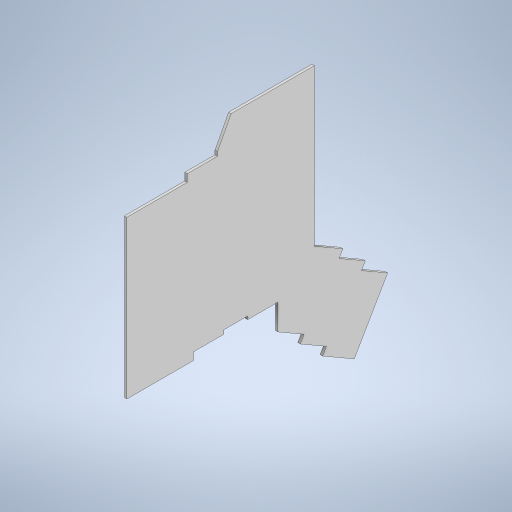
# Autodesk Inventor part: board-profile
Saved by Autodesk Inventor 2024.1 (Build 281209000, 209)
## iProperties
Created: 2023-11-07
Part Number: board-profile
Material: Générique
Document SubType Name: Modeling
Designer: Thibault
Density: 1 g/cm^3
Appearance: Par défaut
Author: Thibault
Autodesk Inventor part; units mm, degrees
ref_plane "YZ Plane" through (0, 0, 0) normal (1, 0, 0) x (0, 1, 0)
ref_plane "XZ Plane" through (0, 0, 0) normal (0, 1, 0) x (-1, 0, 0)
ref_plane "XY Plane" through (0, 0, 0) normal (0, 0, 1) x (1, 0, 0)
sketch "Key" plane through (0, 0, 0) normal (0, 0, 1) x (1, 0, 0)
  line L0 (-9.525, 9.525) -> (9.525, 9.525) construction
  line L1 (9.525, 9.525) -> (9.525, -9.525) construction
  line L2 (9.525, -9.525) -> (-9.525, -9.525) construction
  line L3 (-9.525, -9.525) -> (-9.525, 9.525) construction
  line L4 (-9.525, 9.525) -> (9.525, -9.525) construction
  line L5 (9.525, 9.525) -> (-9.525, -9.525) construction
  point P0 (0, 0)
  point P1 (0, 0)
  dimension "d6" = 19.05
  dimension "d7" = 19.05
  measures "d6" distance of L1.end L2.end
  measures "d7" distance of L0.end L1.end
sketch "Col5" plane through (0, 0, 0) normal (0, 0, 1) x (1, 0, 0)
  line L0 (8.1849, 9.525) -> (27.2349, 9.525) construction
  line L1 (27.2349, 9.525) -> (27.2349, -9.525) construction
  line L2 (27.2349, -9.525) -> (8.1849, -9.525) construction
  line L3 (8.1849, -9.525) -> (8.1849, 9.525) construction
  line L4 (8.1849, 9.525) -> (27.2349, -9.525) construction
  line L5 (27.2349, 9.525) -> (8.1849, -9.525) construction
  line L6 (-10.8651, 9.525) -> (8.1849, 9.525) construction
  line L7 (8.1849, 9.525) -> (8.1849, -9.525) construction
  line L8 (8.1849, -9.525) -> (-10.8651, -9.525) construction
  line L9 (-10.8651, -9.525) -> (-10.8651, 9.525) construction
  line L10 (-10.8651, 9.525) -> (8.1849, -9.525) construction
  line L11 (8.1849, 9.525) -> (-10.8651, -9.525) construction
  line L12 (-29.9151, 9.525) -> (-10.8651, 9.525) construction
  line L13 (-10.8651, 9.525) -> (-10.8651, -9.525) construction
  line L14 (-10.8651, -9.525) -> (-29.9151, -9.525) construction
  line L15 (-29.9151, -9.525) -> (-29.9151, 9.525) construction
  line L16 (-29.9151, 9.525) -> (-10.8651, -9.525) construction
  line L17 (-10.8651, 9.525) -> (-29.9151, -9.525) construction
  line L18 (-48.9651, 9.525) -> (-29.9151, 9.525) construction
  line L19 (-29.9151, 9.525) -> (-29.9151, -9.525) construction
  line L20 (-29.9151, -9.525) -> (-48.9651, -9.525) construction
  line L21 (-48.9651, -9.525) -> (-48.9651, 9.525) construction
  line L22 (-48.9651, 9.525) -> (-29.9151, -9.525) construction
  line L23 (-29.9151, 9.525) -> (-48.9651, -9.525) construction
  line L24 (27.2349, 9.525) -> (46.2849, 9.525) construction
  line L25 (46.2849, 9.525) -> (46.2849, -9.525) construction
  line L26 (46.2849, -9.525) -> (27.2349, -9.525) construction
  line L27 (27.2349, -9.525) -> (27.2349, 9.525) construction
  line L28 (27.2349, 9.525) -> (46.2849, -9.525) construction
  line L29 (46.2849, 9.525) -> (27.2349, -9.525) construction
  point P0 (-10.8651, 0)
sketch "Col4" plane through (0, 0, 0) normal (0, 0, 1) x (1, 0, 0)
  line L0 (8.1849, 9.525) -> (27.2349, 9.525) construction
  line L1 (27.2349, 9.525) -> (27.2349, -9.525) construction
  line L2 (27.2349, -9.525) -> (8.1849, -9.525) construction
  line L3 (8.1849, -9.525) -> (8.1849, 9.525) construction
  line L4 (8.1849, 9.525) -> (27.2349, -9.525) construction
  line L5 (27.2349, 9.525) -> (8.1849, -9.525) construction
  line L6 (-10.8651, 9.525) -> (8.1849, 9.525) construction
  line L7 (8.1849, 9.525) -> (8.1849, -9.525) construction
  line L8 (8.1849, -9.525) -> (-10.8651, -9.525) construction
  line L9 (-10.8651, -9.525) -> (-10.8651, 9.525) construction
  line L10 (-10.8651, 9.525) -> (8.1849, -9.525) construction
  line L11 (8.1849, 9.525) -> (-10.8651, -9.525) construction
  line L12 (-29.9151, 9.525) -> (-10.8651, 9.525) construction
  line L13 (-10.8651, 9.525) -> (-10.8651, -9.525) construction
  line L14 (-10.8651, -9.525) -> (-29.9151, -9.525) construction
  line L15 (-29.9151, -9.525) -> (-29.9151, 9.525) construction
  line L16 (-29.9151, 9.525) -> (-10.8651, -9.525) construction
  line L17 (-10.8651, 9.525) -> (-29.9151, -9.525) construction
  line L18 (-48.9651, 9.525) -> (-29.9151, 9.525) construction
  line L19 (-29.9151, 9.525) -> (-29.9151, -9.525) construction
  line L20 (-29.9151, -9.525) -> (-48.9651, -9.525) construction
  line L21 (-48.9651, -9.525) -> (-48.9651, 9.525) construction
  line L22 (-48.9651, 9.525) -> (-29.9151, -9.525) construction
  line L23 (-29.9151, 9.525) -> (-48.9651, -9.525) construction
  point P0 (-10.8651, 0)
sketch "TC" plane through (0, 0, 0) normal (0, 0, 1) x (1, 0, 0)
  line L0 (-14.8187, 190.1917) -> (1.679, 180.6667) construction
  line L1 (1.679, 180.6667) -> (-7.846, 164.1689) construction
  line L2 (-7.846, 164.1689) -> (-24.3437, 173.6939) construction
  line L3 (-24.3437, 173.6939) -> (-14.8187, 190.1917) construction
  line L4 (-14.8187, 190.1917) -> (-7.846, 164.1689) construction
  line L5 (1.679, 180.6667) -> (-24.3437, 173.6939) construction
  line L6 (-31.3165, 199.7167) -> (-14.8187, 190.1917) construction
  line L7 (-14.8187, 190.1917) -> (-24.3437, 173.6939) construction
  line L8 (-24.3437, 173.6939) -> (-40.8415, 183.2189) construction
  line L9 (-40.8415, 183.2189) -> (-31.3165, 199.7167) construction
  line L10 (-31.3165, 199.7167) -> (-24.3437, 173.6939) construction
  line L11 (-14.8187, 190.1917) -> (-40.8415, 183.2189) construction
  line L12 (-28.4682, 176.0751) -> (-11.9704, 166.5501) construction
  line L13 (-11.9704, 166.5501) -> (-21.4954, 150.0524) construction
  line L14 (-21.4954, 150.0524) -> (-37.9932, 159.5774) construction
  line L15 (-37.9932, 159.5774) -> (-28.4682, 176.0751) construction
  line L16 (-28.4682, 176.0751) -> (-21.4954, 150.0524) construction
  line L17 (-11.9704, 166.5501) -> (-37.9932, 159.5774) construction
  line L18 (-44.966, 185.6001) -> (-28.4682, 176.0751) construction
  line L19 (-28.4682, 176.0751) -> (-37.9932, 159.5774) construction
  line L20 (-37.9932, 159.5774) -> (-54.491, 169.1024) construction
  line L21 (-54.491, 169.1024) -> (-44.966, 185.6001) construction
  line L22 (-44.966, 185.6001) -> (-37.9932, 159.5774) construction
  line L23 (-28.4682, 176.0751) -> (-54.491, 169.1024) construction
  line L24 (-42.1176, 161.9586) -> (-25.6199, 152.4336) construction
  line L25 (-25.6199, 152.4336) -> (-35.1449, 135.9358) construction
  line L26 (-35.1449, 135.9358) -> (-51.6426, 145.4608) construction
  line L27 (-51.6426, 145.4608) -> (-42.1176, 161.9586) construction
  line L28 (-42.1176, 161.9586) -> (-35.1449, 135.9358) construction
  line L29 (-25.6199, 152.4336) -> (-51.6426, 145.4608) construction
  line L30 (-58.6154, 171.4836) -> (-42.1176, 161.9586) construction
  line L31 (-42.1176, 161.9586) -> (-51.6426, 145.4608) construction
  line L32 (-51.6426, 145.4608) -> (-68.1404, 154.9858) construction
  line L33 (-68.1404, 154.9858) -> (-58.6154, 171.4836) construction
  line L34 (-58.6154, 171.4836) -> (-51.6426, 145.4608) construction
  line L35 (-42.1176, 161.9586) -> (-68.1404, 154.9858) construction
  point P0 (-22.1335, 152.0917)
  dimension "d12" = 4.7625
  dimension "d13" = 4.7625
  dimension "d14" = 19.6363
sketch "Esquisse1" plane through (0, 0, 0) normal (1, 0, 0) x (0, 1, 0)
  line L0 (28.177, -71.755) -> (10.397, -71.755) construction
  line L1 (10.397, -71.755) -> (10.397, -102.235) construction
  line L2 (10.397, -102.235) -> (28.177, -102.235)
  line L3 (28.177, -102.235) -> (28.177, -71.755) construction
  line L4 (28.177, -71.755) -> (10.397, -102.235) construction
  line L5 (10.397, -71.755) -> (28.177, -102.235) construction
  line L6 (6.445, 14.065) -> (-92.805, 14.065)
  line L7 (6.445, 14.065) -> (6.445, -24.035)
  line L8 (-68.4861, -104.235) -> (30.177, -104.235)
  line L9 (30.177, -51.755) -> (30.177, -104.235)
  line L10 (-106.1694, -150.4545) -> (-142.6291, -129.4045)
  line L11 (-103.8052, -81.2096) -> (-113.3302, -97.7073)
  line L12 (-113.3302, -97.7073) -> (-117.4547, -95.3261)
  line L13 (-117.4547, -95.3261) -> (-126.9797, -111.8239)
  line L14 (-126.9797, -111.8239) -> (-131.1041, -109.4426)
  line L15 (-131.1041, -109.4426) -> (-142.6291, -129.4045)
  line L16 (-68.4861, -104.235) -> (-78.8706, -122.2214)
  line L17 (-78.8706, -122.2214) -> (-82.995, -119.8402)
  line L18 (-82.995, -119.8402) -> (-92.52, -136.338)
  line L19 (-92.52, -136.338) -> (-96.6444, -133.9567)
  line L20 (-96.6444, -133.9567) -> (-106.1694, -150.4545)
  line L21 (-92.805, 14.065) -> (-92.805, -28.035)
  line L22 (-92.805, -28.035) -> (-88.042, -28.035)
  line L23 (-88.042, -28.035) -> (-88.042, -47.085)
  line L24 (-88.042, -47.085) -> (-85.565, -47.085)
  line L25 (-85.565, -47.085) -> (-85.565, -62.135)
  line L26 (-85.565, -62.135) -> (-87.565, -62.135)
  line L27 (-89.5164, -89.4592) -> (-103.8052, -81.2096) construction
  line L28 (6.445, -24.035) -> (11.208, -24.035)
  line L29 (11.208, -24.035) -> (11.208, -43.085)
  line L30 (11.208, -43.085) -> (13.685, -43.085)
  line L31 (30.177, -51.755) -> (13.685, -43.085)
  line L32 (-78.8706, -122.2214) -> (-92.52, -136.338) construction
  line L33 (-92.52, -136.338) -> (-106.1694, -150.4545) construction
  line L34 (-103.8052, -81.2096) -> (-117.4547, -95.3261) construction
  line L35 (-131.1041, -109.4426) -> (-117.4547, -95.3261) construction
  line L36 (-103.8052, -81.2096) -> (-87.565, -81.2096)
  line L37 (-87.565, -81.2096) -> (-87.565, -62.135)
  line L38 (-33.655, 12.065) -> (-14.605, 12.065) construction
  line L39 (-14.605, 12.065) -> (-14.605, -6.985) construction
  line L40 (-14.605, -6.985) -> (-33.655, -6.985) construction
  line L41 (-33.655, -6.985) -> (-33.655, 12.065) construction
  line L42 (-33.655, 12.065) -> (-14.605, -6.985) construction
  line L43 (-14.605, 12.065) -> (-33.655, -6.985) construction
  line L44 (-52.705, 12.065) -> (-33.655, 12.065) construction
  line L45 (-33.655, 12.065) -> (-33.655, -6.985) construction
  line L46 (-33.655, -6.985) -> (-52.705, -6.985) construction
  line L47 (-52.705, -6.985) -> (-52.705, 12.065) construction
  line L48 (-52.705, 12.065) -> (-33.655, -6.985) construction
  line L49 (-33.655, 12.065) -> (-52.705, -6.985) construction
  line L50 (-71.755, 12.065) -> (-52.705, 12.065) construction
  line L51 (-52.705, 12.065) -> (-52.705, -6.985) construction
  line L52 (-52.705, -6.985) -> (-71.755, -6.985) construction
  line L53 (-71.755, -6.985) -> (-71.755, 12.065) construction
  line L54 (-71.755, 12.065) -> (-52.705, -6.985) construction
  line L55 (-52.705, 12.065) -> (-71.755, -6.985) construction
  line L56 (-90.805, 12.065) -> (-71.755, 12.065) construction
  line L57 (-71.755, 12.065) -> (-71.755, -6.985) construction
  line L58 (-71.755, -6.985) -> (-90.805, -6.985) construction
  line L59 (-90.805, -6.985) -> (-90.805, 12.065) construction
  line L60 (-90.805, 12.065) -> (-71.755, -6.985) construction
  line L61 (-71.755, 12.065) -> (-90.805, -6.985) construction
  line L62 (-14.605, 12.065) -> (4.445, 12.065) construction
  line L63 (4.445, 12.065) -> (4.445, -6.985) construction
  line L64 (4.445, -6.985) -> (-14.605, -6.985) construction
  line L65 (-14.605, -6.985) -> (-14.605, 12.065) construction
  line L66 (-14.605, 12.065) -> (4.445, -6.985) construction
  line L67 (4.445, 12.065) -> (-14.605, -6.985) construction
  line L68 (-33.655, -6.985) -> (-14.605, -6.985) construction
  line L69 (-14.605, -6.985) -> (-14.605, -26.035) construction
  line L70 (-14.605, -26.035) -> (-33.655, -26.035) construction
  line L71 (-33.655, -26.035) -> (-33.655, -6.985) construction
  line L72 (-33.655, -6.985) -> (-14.605, -26.035) construction
  line L73 (-14.605, -6.985) -> (-33.655, -26.035) construction
  line L74 (-52.705, -6.985) -> (-33.655, -6.985) construction
  line L75 (-33.655, -6.985) -> (-33.655, -26.035) construction
  line L76 (-33.655, -26.035) -> (-52.705, -26.035) construction
  line L77 (-52.705, -26.035) -> (-52.705, -6.985) construction
  line L78 (-52.705, -6.985) -> (-33.655, -26.035) construction
  line L79 (-33.655, -6.985) -> (-52.705, -26.035) construction
  line L80 (-71.755, -6.985) -> (-52.705, -6.985) construction
  line L81 (-52.705, -6.985) -> (-52.705, -26.035) construction
  line L82 (-52.705, -26.035) -> (-71.755, -26.035) construction
  line L83 (-71.755, -26.035) -> (-71.755, -6.985) construction
  line L84 (-71.755, -6.985) -> (-52.705, -26.035) construction
  line L85 (-52.705, -6.985) -> (-71.755, -26.035) construction
  line L86 (-90.805, -6.985) -> (-71.755, -6.985) construction
  line L87 (-71.755, -6.985) -> (-71.755, -26.035) construction
  line L88 (-71.755, -26.035) -> (-90.805, -26.035) construction
  line L89 (-90.805, -26.035) -> (-90.805, -6.985) construction
  line L90 (-90.805, -6.985) -> (-71.755, -26.035) construction
  line L91 (-71.755, -6.985) -> (-90.805, -26.035) construction
  line L92 (-14.605, -6.985) -> (4.445, -6.985) construction
  line L93 (4.445, -6.985) -> (4.445, -26.035) construction
  line L94 (4.445, -26.035) -> (-14.605, -26.035) construction
  line L95 (-14.605, -26.035) -> (-14.605, -6.985) construction
  line L96 (-14.605, -6.985) -> (4.445, -26.035) construction
  line L97 (4.445, -6.985) -> (-14.605, -26.035) construction
  line L98 (-28.892, -26.035) -> (-9.842, -26.035) construction
  line L99 (-9.842, -26.035) -> (-9.842, -45.085) construction
  line L100 (-9.842, -45.085) -> (-28.892, -45.085) construction
  line L101 (-28.892, -45.085) -> (-28.892, -26.035) construction
  line L102 (-28.892, -26.035) -> (-9.842, -45.085) construction
  line L103 (-9.842, -26.035) -> (-28.892, -45.085) construction
  line L104 (-47.942, -26.035) -> (-28.892, -26.035) construction
  line L105 (-28.892, -26.035) -> (-28.892, -45.085) construction
  line L106 (-28.892, -45.085) -> (-47.942, -45.085) construction
  line L107 (-47.942, -45.085) -> (-47.942, -26.035) construction
  line L108 (-47.942, -26.035) -> (-28.892, -45.085) construction
  line L109 (-28.892, -26.035) -> (-47.942, -45.085) construction
  line L110 (-66.992, -26.035) -> (-47.942, -26.035) construction
  line L111 (-47.942, -26.035) -> (-47.942, -45.085) construction
  line L112 (-47.942, -45.085) -> (-66.992, -45.085) construction
  line L113 (-66.992, -45.085) -> (-66.992, -26.035) construction
  line L114 (-66.992, -26.035) -> (-47.942, -45.085) construction
  line L115 (-47.942, -26.035) -> (-66.992, -45.085) construction
  line L116 (-86.042, -26.035) -> (-66.992, -26.035) construction
  line L117 (-66.992, -26.035) -> (-66.992, -45.085) construction
  line L118 (-66.992, -45.085) -> (-86.042, -45.085) construction
  line L119 (-86.042, -45.085) -> (-86.042, -26.035) construction
  line L120 (-86.042, -26.035) -> (-66.992, -45.085) construction
  line L121 (-66.992, -26.035) -> (-86.042, -45.085) construction
  line L122 (-9.842, -26.035) -> (9.208, -26.035) construction
  line L123 (9.208, -26.035) -> (9.208, -45.085) construction
  line L124 (9.208, -45.085) -> (-9.842, -45.085) construction
  line L125 (-9.842, -45.085) -> (-9.842, -26.035) construction
  line L126 (-9.842, -26.035) -> (9.208, -45.085) construction
  line L127 (9.208, -26.035) -> (-9.842, -45.085) construction
  line L128 (-26.415, -45.085) -> (-7.365, -45.085) construction
  line L129 (-7.365, -45.085) -> (-7.365, -64.135) construction
  line L130 (-7.365, -64.135) -> (-26.415, -64.135) construction
  line L131 (-26.415, -64.135) -> (-26.415, -45.085) construction
  line L132 (-26.415, -45.085) -> (-7.365, -64.135) construction
  line L133 (-7.365, -45.085) -> (-26.415, -64.135) construction
  line L134 (-45.465, -45.085) -> (-26.415, -45.085) construction
  line L135 (-26.415, -45.085) -> (-26.415, -64.135) construction
  line L136 (-26.415, -64.135) -> (-45.465, -64.135) construction
  line L137 (-45.465, -64.135) -> (-45.465, -45.085) construction
  line L138 (-45.465, -45.085) -> (-26.415, -64.135) construction
  line L139 (-26.415, -45.085) -> (-45.465, -64.135) construction
  line L140 (-64.515, -45.085) -> (-45.465, -45.085) construction
  line L141 (-45.465, -45.085) -> (-45.465, -64.135) construction
  line L142 (-45.465, -64.135) -> (-64.515, -64.135) construction
  line L143 (-64.515, -64.135) -> (-64.515, -45.085) construction
  line L144 (-64.515, -45.085) -> (-45.465, -64.135) construction
  line L145 (-45.465, -45.085) -> (-64.515, -64.135) construction
  line L146 (-83.565, -45.085) -> (-64.515, -45.085) construction
  line L147 (-64.515, -45.085) -> (-64.515, -64.135) construction
  line L148 (-64.515, -64.135) -> (-83.565, -64.135) construction
  line L149 (-83.565, -64.135) -> (-83.565, -45.085) construction
  line L150 (-83.565, -45.085) -> (-64.515, -64.135) construction
  line L151 (-64.515, -45.085) -> (-83.565, -64.135) construction
  line L152 (-7.365, -45.085) -> (11.685, -45.085) construction
  line L153 (11.685, -45.085) -> (11.685, -64.135) construction
  line L154 (11.685, -64.135) -> (-7.365, -64.135) construction
  line L155 (-7.365, -64.135) -> (-7.365, -45.085) construction
  line L156 (-7.365, -45.085) -> (11.685, -64.135) construction
  line L157 (11.685, -45.085) -> (-7.365, -64.135) construction
  line L158 (-28.892, -64.135) -> (-9.842, -64.135) construction
  line L159 (-9.842, -64.135) -> (-9.842, -83.185) construction
  line L160 (-9.842, -83.185) -> (-28.892, -83.185) construction
  line L161 (-28.892, -83.185) -> (-28.892, -64.135) construction
  line L162 (-28.892, -64.135) -> (-9.842, -83.185) construction
  line L163 (-9.842, -64.135) -> (-28.892, -83.185) construction
  line L164 (-47.942, -64.135) -> (-28.892, -64.135) construction
  line L165 (-28.892, -64.135) -> (-28.892, -83.185) construction
  line L166 (-28.892, -83.185) -> (-47.942, -83.185) construction
  line L167 (-47.942, -83.185) -> (-47.942, -64.135) construction
  line L168 (-47.942, -64.135) -> (-28.892, -83.185) construction
  line L169 (-28.892, -64.135) -> (-47.942, -83.185) construction
  line L170 (-66.992, -64.135) -> (-47.942, -64.135) construction
  line L171 (-47.942, -64.135) -> (-47.942, -83.185) construction
  line L172 (-47.942, -83.185) -> (-66.992, -83.185) construction
  line L173 (-66.992, -83.185) -> (-66.992, -64.135) construction
  line L174 (-66.992, -64.135) -> (-47.942, -83.185) construction
  line L175 (-47.942, -64.135) -> (-66.992, -83.185) construction
  line L176 (-86.042, -64.135) -> (-66.992, -64.135) construction
  line L177 (-66.992, -64.135) -> (-66.992, -83.185) construction
  line L178 (-66.992, -83.185) -> (-86.042, -83.185) construction
  line L179 (-86.042, -83.185) -> (-86.042, -64.135) construction
  line L180 (-86.042, -64.135) -> (-66.992, -83.185) construction
  line L181 (-66.992, -64.135) -> (-86.042, -83.185) construction
  line L182 (-9.842, -64.135) -> (9.208, -64.135) construction
  line L183 (9.208, -64.135) -> (9.208, -83.185) construction
  line L184 (9.208, -83.185) -> (-9.842, -83.185) construction
  line L185 (-9.842, -83.185) -> (-9.842, -64.135) construction
  line L186 (-9.842, -64.135) -> (9.208, -83.185) construction
  line L187 (9.208, -64.135) -> (-9.842, -83.185) construction
  line L188 (-12.128, -83.185) -> (6.922, -83.185) construction
  line L189 (6.922, -83.185) -> (6.922, -102.235) construction
  line L190 (6.922, -102.235) -> (-12.128, -102.235) construction
  line L191 (-12.128, -102.235) -> (-12.128, -83.185) construction
  line L192 (-12.128, -83.185) -> (6.922, -102.235) construction
  line L193 (6.922, -83.185) -> (-12.128, -102.235) construction
  line L194 (-31.178, -83.185) -> (-12.128, -83.185) construction
  line L195 (-12.128, -83.185) -> (-12.128, -102.235) construction
  line L196 (-12.128, -102.235) -> (-31.178, -102.235) construction
  line L197 (-31.178, -102.235) -> (-31.178, -83.185) construction
  line L198 (-31.178, -83.185) -> (-12.128, -102.235) construction
  line L199 (-12.128, -83.185) -> (-31.178, -102.235) construction
  line L200 (-50.228, -83.185) -> (-31.178, -83.185) construction
  line L201 (-31.178, -83.185) -> (-31.178, -102.235) construction
  line L202 (-31.178, -102.235) -> (-50.228, -102.235) construction
  line L203 (-50.228, -102.235) -> (-50.228, -83.185) construction
  line L204 (-50.228, -83.185) -> (-31.178, -102.235) construction
  line L205 (-31.178, -83.185) -> (-50.228, -102.235) construction
  line L206 (-69.278, -83.185) -> (-50.228, -83.185) construction
  line L207 (-50.228, -83.185) -> (-50.228, -102.235) construction
  line L208 (-50.228, -102.235) -> (-69.278, -102.235) construction
  line L209 (-69.278, -102.235) -> (-69.278, -83.185) construction
  line L210 (-69.278, -83.185) -> (-50.228, -102.235) construction
  line L211 (-50.228, -83.185) -> (-69.278, -102.235) construction
  line L212 (-86.5754, -93.4666) -> (-70.0776, -102.9916) construction
  line L213 (-70.0776, -102.9916) -> (-79.6026, -119.4894) construction
  line L214 (-79.6026, -119.4894) -> (-96.1004, -109.9644) construction
  line L215 (-96.1004, -109.9644) -> (-86.5754, -93.4666) construction
  line L216 (-86.5754, -93.4666) -> (-79.6026, -119.4894) construction
  line L217 (-70.0776, -102.9916) -> (-96.1004, -109.9644) construction
  line L218 (-103.0732, -83.9416) -> (-86.5754, -93.4666) construction
  line L219 (-86.5754, -93.4666) -> (-96.1004, -109.9644) construction
  line L220 (-96.1004, -109.9644) -> (-112.5982, -100.4394) construction
  line L221 (-112.5982, -100.4394) -> (-103.0732, -83.9416) construction
  line L222 (-103.0732, -83.9416) -> (-96.1004, -109.9644) construction
  line L223 (-86.5754, -93.4666) -> (-112.5982, -100.4394) construction
  line L224 (-100.2248, -107.5831) -> (-83.7271, -117.1081) construction
  line L225 (-83.7271, -117.1081) -> (-93.2521, -133.6059) construction
  line L226 (-93.2521, -133.6059) -> (-109.7498, -124.0809) construction
  line L227 (-109.7498, -124.0809) -> (-100.2248, -107.5831) construction
  line L228 (-100.2248, -107.5831) -> (-93.2521, -133.6059) construction
  line L229 (-83.7271, -117.1081) -> (-109.7498, -124.0809) construction
  line L230 (-116.7226, -98.0581) -> (-100.2248, -107.5831) construction
  line L231 (-100.2248, -107.5831) -> (-109.7498, -124.0809) construction
  line L232 (-109.7498, -124.0809) -> (-126.2476, -114.5559) construction
  line L233 (-126.2476, -114.5559) -> (-116.7226, -98.0581) construction
  line L234 (-116.7226, -98.0581) -> (-109.7498, -124.0809) construction
  line L235 (-100.2248, -107.5831) -> (-126.2476, -114.5559) construction
  line L236 (-113.8743, -121.6997) -> (-97.3765, -131.2247) construction
  line L237 (-97.3765, -131.2247) -> (-106.9015, -147.7225) construction
  line L238 (-106.9015, -147.7225) -> (-123.3993, -138.1975) construction
  line L239 (-123.3993, -138.1975) -> (-113.8743, -121.6997) construction
  line L240 (-113.8743, -121.6997) -> (-106.9015, -147.7225) construction
  line L241 (-97.3765, -131.2247) -> (-123.3993, -138.1975) construction
  line L242 (-130.3721, -112.1747) -> (-113.8743, -121.6997) construction
  line L243 (-113.8743, -121.6997) -> (-123.3993, -138.1975) construction
  line L244 (-123.3993, -138.1975) -> (-139.8971, -128.6725) construction
  line L245 (-139.8971, -128.6725) -> (-130.3721, -112.1747) construction
  line L246 (-130.3721, -112.1747) -> (-123.3993, -138.1975) construction
  line L247 (-113.8743, -121.6997) -> (-139.8971, -128.6725) construction
  point P0 (-5.08, 2.54)
  point P1 (19.287, -86.995)
  point P2 (-5.08, 2.54)
  point P3 (-86.042, -35.56)
  point P4 (0, 0)
extrude "Extrusion1" add sketch "Esquisse1" along normal blind 1.6
